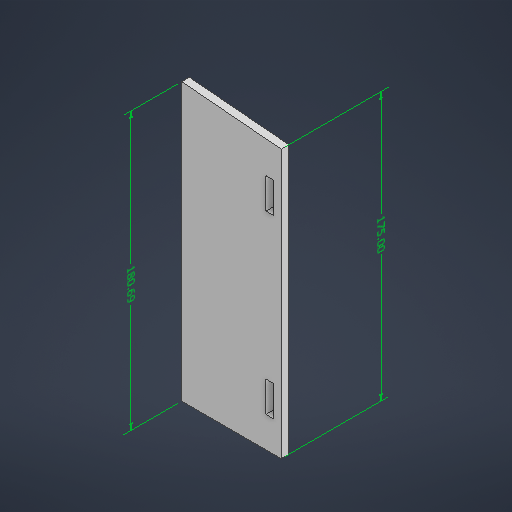
# Autodesk Inventor part: standformiddleslide1
Saved by Autodesk Inventor 2026.2 (Build 302298000, 298)
## iProperties
Created: 2026-02-23
Part Number: standformiddleslide1
Material: Generic
Document SubType Name: Sheet Metal
Designer: danda
Density: 1 g/cm^3
Sheet Metal Rule: Default_mm
Appearance: Default
Author: danda
Autodesk Inventor part; units mm, degrees
ref_plane "YZ Plane" through (0, 0, 0) normal (1, 0, 0) x (0, 1, 0)
ref_plane "XZ Plane" through (0, 0, 0) normal (0, 1, 0) x (-1, 0, 0)
ref_plane "XY Plane" through (0, 0, 0) normal (0, 0, 1) x (1, 0, 0)
sketch "Sketch1" plane through (0, 0, 0) normal (0, 0, 1) x (1, 0, 0)
  line L0 (14.1765, -19.066) -> (14.1765, 161.6208)
  line L1 (14.1765, -19.066) -> (79.1765, -19.066)
  line L2 (79.1765, -19.066) -> (79.1765, 155.934)
  line L3 (79.1765, -19.066) -> (14.1765, -19.066)
  line L4 (79.1765, -19.066) -> (14.1765, -19.066)
  line L5 (14.1765, 161.6208) -> (79.1765, 155.934)
  line L6 (79.1765, 135.934) -> (74.1765, 135.934)
  line L7 (74.1765, 135.934) -> (74.1765, 115.934)
  line L8 (74.1765, 115.934) -> (79.1765, 115.934)
  line L9 (79.1765, 115.934) -> (79.1765, 135.934)
  line L10 (69.1765, 20.934) -> (74.1765, 20.934)
  line L11 (74.1765, 20.934) -> (74.1765, 0.934)
  line L12 (74.1765, 0.934) -> (69.1765, 0.934)
  line L13 (69.1765, 0.934) -> (69.1765, 20.934)
  line L14 (74.1765, 135.934) -> (69.1765, 135.934)
  line L15 (69.1765, 135.934) -> (69.1765, 115.934)
  line L16 (69.1765, 115.934) -> (74.1765, 115.934)
  line L17 (74.1765, 115.934) -> (74.1765, 135.934)
  point P0 (0, 0)
  point P1 (71.6765, 0.934)
  point P2 (79.2985, 0.69)
  point P3 (79.2985, 20.69)
  point P4 (79.1765, 115.934)
  dimension "d3" = 65
  dimension "d23" = 85
  dimension "d26" = 175
  dimension "d27" = 180.6868
  dimension "d28" = 5
  dimension "d29" = 20
  dimension "d30" = 5
  dimension "d31" = 20
  dimension "d32" = 20
  dimension "d33" = 20
  dimension "d35" = 5
  dimension "d36" = 5
  constraints: 36 end point, 6 parallel, 4 perpendicular, 3 horizontal, 2 vertical, 1 midpoint, 1 point on line
  measures "d3" distance of L0.start L1.end
  measures "d23" angle of L0 L5
  measures "d26" distance of L1.end L2.end
  measures "d27" distance of L0.start L0.end
  measures "d28" distance of L8.end L7.end
  measures "d29" distance of L7.end L6.end
  measures "d30" distance of L11.end L12.end
  measures "d31" distance of L10.end L11.end
  measures "d32" distance from line of L2.end L6
  measures "d33" vertical distance of L1.end point (71.676, 0.934)
  measures "d35" distance between parallel lines of L11 L2
  measures "d36" distance of L16.end L15.end
extrude "Extrusion1" add sketch "Sketch1" along normal mid plane 5 contours L0 L5 L2 L6 L14 L15 L16 L8 L1 | L8 L7 L6 L2
equation "\"BendRadius\" = Thickness"
equation "\"BendReliefWidth\" = Thickness"
equation "\"BendReliefDepth\" = 0.5 * Thickness"
equation "\"CornerReliefSize\" = 4 * Thickness"
equation "\"MinimumRemnant\" = 2 * Thickness"
equation "\"TransitionRadius\" = BendRadius"
equation "\"JacobiRadiusSize\" = BendRadius"
equation "\"GapSize\" = Thickness"
equation "\"Thickness\" = 0.5"
body "Solid1"
